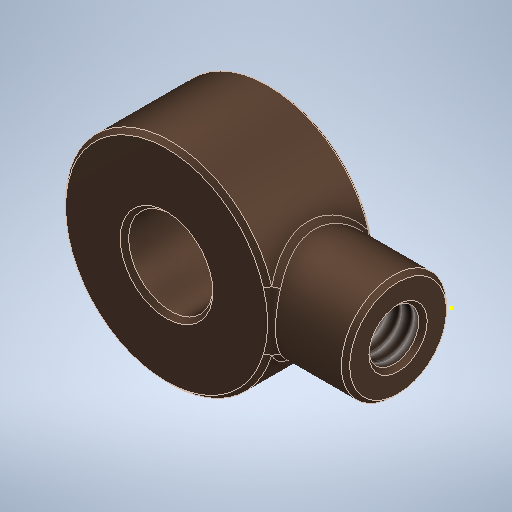
# Autodesk Inventor part: 25 - Disc Arm 1
Saved by Autodesk Inventor 2025.2 (Build 292293000, 293)
## iProperties
Created: 2025-07-17
Part Number: 25 - Disc Arm 1
Material: Bronze, Soft Tin
Document SubType Name: Modeling
Designer: bless
Density: 8.874 g/cm^3
Appearance: Bronze - Satin
Author: bless
Autodesk Inventor part; units mm, degrees
ref_plane "XZ Plane" through (0, 0, 0) normal (0, 1, 0) x (-1, 0, 0)
ref_plane "XY Plane" through (0, 0, 0) normal (0, 0, 1) x (1, 0, 0)
sketch "Sketch1" plane through (0, 0, 0) normal (0, 0, 1) x (1, 0, 0)
  circle A0 centre (0, 0) radius 1
  circle A1 centre (0, 0) radius 2.5
  dimension "d0" = 2
  dimension "d1" = 2.5
  constraints: 2 centre point, 2 coincident
  measures "d0" diameter of A0
  measures "d1" radius of A1
extrude "Extrusion1" add sketch "Sketch1" along normal blind 2.5
ref_plane "Work Plane1" through (4.25, 0, 0) normal (1, 0, 0) x (0, 1, 0)
sketch "Sketch2" plane through (4.25, 0, 0) normal (1, 0, 0) x (0, 1, 0)
  point P0 (0, 0)
sketch "Sketch3" plane through (4.25, 0, 0) normal (1, 0, 0) x (0, 1, 0)
  line L0 (2.5, 0) -> (2.5, 2.5) projected
  line L1 (-2.5, 0) -> (-2.5, 2.5) projected
  line L2 (2.5, 2.5) -> (-2.5, 2.5) projected
  line L3 (2.5, 0) -> (-2.5, 0) projected
  circle A0 centre (0, 1.25) radius 1.25
  point P0 (0, 0)
  constraints: 2 horizontal, 1 vertical alignment, 2 other
extrude "Extrusion2" add sketch "Sketch3" against normal up to surface contours A0
sketch "Sketch4" plane through (4.25, 0, 1.25) normal (1, 0, 0) x (0, 0, -1)
  circle A0 centre (0, 0) radius 1.25 projected
  point P0 (1.25, 0)
  constraints: 1 horizontal alignment
hole "Hole1" at (4.25, 0, 1.25) direction (-1, 0, 0) diameter 1.1835 depth 2.4 tip angle 118 thread size "M1.4x0.3" class "6H" standard "ANSI Metric M Profile"
chamfer "Chamfer1" distance 0.1 angle 45 10 edges at (-2.5, 0, 0) (4.25, -1.25, 1.25) (1.85, 0, 1.8417) (4.25, 0, 1.8417) (-2.5, 0, 2.5) (2.1651, -1.25, 1.25) (2.3231, 0.9237, 2.0922) (2.3231, 0.9237, 0.4078) (-1, 0, 0) (-1, 0, 2.5)
body "Solid1"
